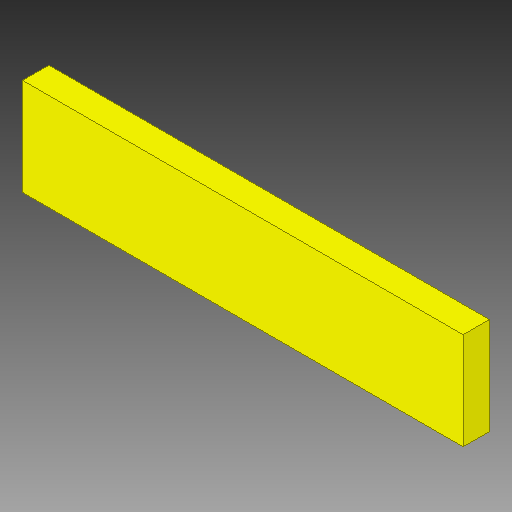
# Autodesk Inventor part: U_1_LOGO16_TPLACE
Saved by Autodesk Inventor 2018 (Build 220112000, 112)
## iProperties
Created: 2015-11-24
Part Number: U_1_LOGO16_TPLACE
Material: Generic
Document SubType Name: Modeling
Designer: PhillipD
Density: 1 g/cm^3
Appearance: LOGO16_TPLACE, U_1_LOGO16_TPLACE
Author: PhillipD
Autodesk Inventor part; units mm, degrees
ref_plane "YZ Plane" through (0, 0, 0) normal (1, 0, 0) x (0, 1, 0)
ref_plane "XZ Plane" through (0, 0, 0) normal (0, 1, 0) x (-1, 0, 0)
ref_plane "XY Plane" through (0, 0, 0) normal (0, 0, 1) x (1, 0, 0)
sketch "LOGO16_TPLACE, U_1_LOGO16_TPLACE_154" plane through (0, 0, 0) normal (0, 0, 1) x (1, 0, 0)
  line L0 (0, 3.692) -> (16.756, 3.692)
  line L1 (16.756, 3.692) -> (16.756, 0)
  line L2 (16.756, 0) -> (0, 0)
  line L3 (0, 0) -> (0, 3.692)
  constraints: 8 end point
extrude "Extrusion1" add sketch "LOGO16_TPLACE, U_1_LOGO16_TPLACE_154" along normal blind 1
body "Solid1"
